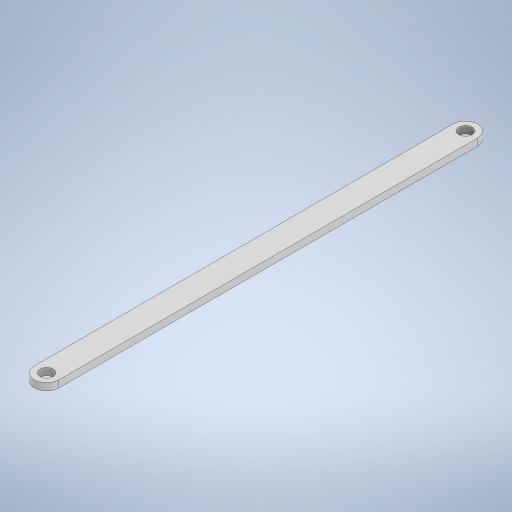
# Autodesk Inventor part: belka
Saved by Autodesk Inventor 2023 (Build 270158000, 158)
## iProperties
Created: 2024-03-30
Part Number: belka
Material: Ogólny
Document SubType Name: Modeling
Designer: Kamil
Density: 1 g/cm^3
Appearance: Domyślna
Author: Kamil
Autodesk Inventor part; units mm, degrees
ref_plane "YZ Plane" through (0, 0, 0) normal (1, 0, 0) x (0, 1, 0)
ref_plane "XZ Plane" through (0, 0, 0) normal (0, 1, 0) x (-1, 0, 0)
ref_plane "XY Plane" through (0, 0, 0) normal (0, 0, 1) x (1, 0, 0)
sketch "Szkic1" plane through (0, 0, 0) normal (0, 1, 0) x (-1, 0, 0)
  line L0 (3.5, 84) -> (-2, 84)
  line L1 (-2, 84) -> (-2, -16)
  line L2 (-2, -16) -> (3.5, -16)
  line L3 (3.5, -16) -> (3.5, 84)
  point P0 (0, 0)
  dimension "d0" = 5.5
  dimension "d1" = 100
  constraints: 8 end point, 2 parallel, 1 horizontal, 1 perpendicular
  measures "d0" distance of L2.end L1.end
  measures "d1" distance of L0.end L1.end
extrude "Wyciągnięcie proste1" add sketch "Szkic1" along normal blind 1.6
fillet "Zaokrąglenie1" radius 2.75 4 edges at (-3.5, 0.8, -16) (2, 0.8, -16) (-3.5, 0.8, 84) (2, 0.8, 84)
sketch "Szkic2" plane through (0, 1.6, 0) normal (0, 1, 0) x (1, 0, 0)
  arc A0 (-3.5, -81.25) -> (2, -81.25) centre (-0.75, -81.25) ccw projected
  line L0 (2, -81.25) -> (2, 13.25) projected
  arc A1 (2, 13.25) -> (-3.5, 13.25) centre (-0.75, 13.25) ccw projected
  line L1 (-3.5, 13.25) -> (-3.5, -81.25) projected
  point P0 (0, 0)
  constraints: 2 coincident
hole "Otwór1" at (-0.75, 1.6, 81.25) at (-0.75, 1.6, -13.25) direction (0, -1, 0) diameter 3 end through all
